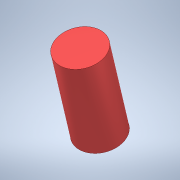
# Autodesk Inventor part: motor
Saved by Autodesk Inventor 2022 (Build 260153070, 153G)
## iProperties
Created: 2021-05-15
Part Number: motor
Material: Aluminum 6061
Document SubType Name: Modeling
Designer: kardo
Density: 2.7 g/cm^3
Appearance: Aluminum - Flat
Mass: 120 g
Surface Area: 61.5752 cm^2
Volume: 34.4821 cm^3
Author: kardo
Autodesk Inventor part; units mm, degrees
ref_plane "YZ Plane" through (0, 0, 0) normal (1, 0, 0) x (0, 1, 0)
ref_plane "XZ Plane" through (0, 0, 0) normal (0, 1, 0) x (-1, 0, 0)
ref_plane "XY Plane" through (0, 0, 0) normal (0, 0, 1) x (1, 0, 0)
derived "powertrain_outline.ipt"
sketch "sk_powertrain" plane through (6.24, 0, 0) normal (1, 0, 0) x (0, 1, 0)
  line L0 (-37.9005, 25.6108) -> (-277.6703, 19.7906) construction
  line L1 (-363, 18.496) -> (-297.6664, 19.4083) construction
  line L2 (94.8, 28.832) -> (28.4595, 27.2216) construction
  line L3 (28.4595, 27.2216) -> (-37.9005, 25.6108) construction
  line L4 (-481.4814, 0) -> (195.5686, 0) construction
  line L5 (-388, 0) -> (-328.1462, 4.1854)
  line L6 (-240.9836, 17.5003) -> (-155.2, 37.8904)
  arc A0 (-328.1462, 4.1854) -> (-240.9836, 17.5003) centre (-365.7957, 542.5994) ccw
  line L7 (-363, 18.496) -> (-388, 18.496) construction
  line L8 (-388, 18.496) -> (-388, 0) construction
  line L9 (-328.1462, 4.1854) -> (-155.2, 16.279) construction
  line L10 (-155.2, 37.8904) -> (-155.2, 16.279) construction
  line L11 (-240.9836, 17.5003) -> (-240.9836, 10.2804) construction
  line L12 (-158.4375, 51.5109) -> (-151.9625, 24.2699)
  line L13 (-151.9625, 24.2699) -> (-97.4804, 37.2199)
  line L14 (-97.4804, 37.2199) -> (-103.9554, 64.4609)
  line L15 (-103.9554, 64.4609) -> (-158.4375, 51.5109)
  line L16 (-158.4375, 51.5109) -> (-97.4804, 37.2199) construction
  line L17 (-151.9625, 24.2699) -> (-103.9554, 64.4609) construction
  line L18 (-151.9625, 24.2699) -> (-151.9625, 19.2699) construction
  line L19 (-328.1462, 4.1854) -> (-240.9836, 17.5003) construction
  spline S0 degree 3 poles (-297.6664, 19.4083) (-291.0004, 19.5014) (-284.3349, 19.6288) (-277.6703, 19.7906) knots 0 0 0 0 1 1 1 1 construction
  spline S1 degree 4 poles (-297.6664, 19.4083) (-178.2238, 21.0761) (-46.6271, 18.3209) (53.0846, 11.363) (94.8, 28.832) knots 0 0 0 0 0 1 1 1 1 1 construction
  spline S2 degree 2 poles (0, 55.974) (-217.9618, 52.7695) (-363, 39.654) knots 0 0 0 1 1 1 construction
  spline S3 degree 4 poles (0, 55.974) (21.4177, 56.2889) (38.251, 53.3044) (69.464, 45.4203) (94.8, 37.536) knots 0 0 0 0 0 1 1 1 1 1 construction
  point P0 (0, 0)
  point P1 (-127.959, 44.3654)
  point P2 (-127.959, 44.3654)
ref_plane "Work Plane1" through (6.24, -155.2, 37.8904) normal (0, 0.9728944, 0.2312497) x (-1, 0, 0)
sketch "Sketch2" plane through (6.24, -155.2, 37.8904) normal (0, 0.9728944, 0.2312497) x (-1, 0, 0)
  circle A0 centre (0, 0) radius 14
  point P0 (6.24, -72.7533)
  dimension "d1" = 28
  constraints: 1 centre point, 1 coincident
  measures "d1" diameter of A0
extrude "Extrusion1" add sketch "Sketch2" along normal blind 56
equation "\"d1\" = motor_diameter"
equation "\"d4\" = motor_length"
equation "\"motor_diameter\" = 28"
equation "\"motor_length\" = 56"
body "Solid1"
